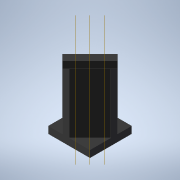
# Autodesk Inventor part: HC-SR04-support
Saved by Autodesk Inventor 2022 (Build 260153000, 153)
## iProperties
Created: 2023-01-18
Part Number: HC-SR04-support
Material: Generic
Document SubType Name: Modeling
Designer: CLCK
Density: 1 g/cm^3
Appearance: Default
Author: CLCK
Autodesk Inventor part; units mm, degrees
ref_plane "YZ Plane" through (0, 0, 0) normal (1, 0, 0) x (0, 1, 0)
ref_plane "XZ Plane" through (0, 0, 0) normal (0, 1, 0) x (-1, 0, 0)
ref_plane "XY Plane" through (0, 0, 0) normal (0, 0, 1) x (1, 0, 0)
sketch "Sketch1" plane through (0, 0, 0) normal (0, 1, 0) x (-1, 0, 0)
  line L0 (10, 0) -> (-20, 0)
  line L1 (-20, 0) -> (-20, 30)
  line L2 (-20, 30) -> (10, 30)
  line L3 (10, 30) -> (10, 0)
  circle A0 centre (0, 10) radius 2
  point P0 (0, 0)
  dimension "d0" = 30
  dimension "d1" = 30
  dimension "d2" = 4
  constraints: 8 end point, 2 parallel, 1 centre point, 1 horizontal, 1 perpendicular
  measures "d0" distance of L1.end L2.end
  measures "d1" distance of L0.end L1.end
  measures "d2" diameter of A0
extrude "Extrusion1" add sketch "Sketch1" along normal blind 5
sketch "Sketch2" plane through (0, 5, 0) normal (0, 1, 0) x (1, 0, 0)
  line L0 (-10, -30) -> (20, -30) projected
  line L1 (5, -30) -> (20, -15)
  line L2 (20, -30) -> (20, 0) projected
  line L3 (0, -30) -> (20, -10)
  line L4 (0, -30) -> (5, -30)
  line L5 (20, -15) -> (20, -10)
  point P0 (0, 0)
  constraints: 8 end point, 2 collinear, 2 midpoint, 1 parallel
extrude "Extrusion2" add sketch "Sketch2" along normal blind 50 contours L3 L2 L1 L0
ref_plane "Work Plane1" through (-10, 0, 0) normal (0.7071068, 0, -0.7071068) x (0, 1, 0)
ref_plane "Work Plane2" through (-4.6967, 0, -5.3033) normal (0.7071068, 0, -0.7071068) x (0, 1, 0)
ref_plane "Work Plane3" through (-15.3033, 0, 5.3033) normal (0.7071068, 0, -0.7071068) x (0, 1, 0)
sketch "Sketch3" plane through (-4.6967, 0, -5.3033) normal (0.7071068, 0, -0.7071068) x (0, 1, 0)
  line L0 (5, 21.2132) -> (5, 28.2843) projected
  line L1 (5, 28.2843) -> (5, 21.2132)
  line L2 (5, 21.2132) -> (16.4907, 28.2843)
  line L3 (5, 28.2843) -> (55, 28.2843) projected
  line L4 (16.4907, 28.2843) -> (5, 28.2843)
  point P0 (0, 7.0711)
  constraints: 6 end point, 2 collinear, 1 point on line
sketch "Sketch4" plane through (-15.3033, 0, 5.3033) normal (0.7071068, 0, -0.7071068) x (0, 1, 0)
  line L0 (5, 20.039) -> (18.3988, 28.2843) projected
  line L1 (5, 28.2843) -> (5, 21.2132) projected
  line L2 (5, 20.039) -> (5, 28.2843)
  line L3 (5, 28.2843) -> (18.2878, 28.2843)
  line L4 (5, 28.2843) -> (55, 28.2843) projected
  point P0 (0, 7.0711)
  point P1 (5, 21.2132)
  constraints: 4 end point, 1 collinear, 1 point on line
extrude "Extrusion3" add sketch "Sketch3" along normal mid plane 2
extrude "Extrusion4" add sketch "Sketch4" along normal mid plane 2
sketch "Sketch5" plane through (0, 5, 30) normal (-0.7071068, 0, -0.7071068) x (-0.7071068, 0, 0.7071068)
  line L0 (0, 0) -> (0, 50) projected
  line L1 (-28.2843, 0) -> (-28.2843, 50) projected
  line L2 (0, 50) -> (-28.2843, 50)
  line L3 (-28.2843, 50) -> (-28.2843, 45)
  line L4 (-28.2843, 45) -> (0, 45)
  line L5 (0, 45) -> (0, 50)
  point P0 (-21.2132, -5)
  dimension "d19" = 5
  constraints: 8 end point, 2 parallel, 1 horizontal, 1 perpendicular, 1 point on line
  measures "d19" distance of L3.end L2.end
extrude "Extrusion5" add sketch "Sketch5" against normal blind 6
body "Solid1"
